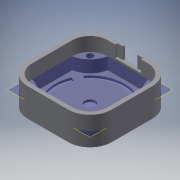
# Autodesk Inventor part: Oberbau
Saved by Autodesk Inventor 2018 (Build 220112000, 112)
## iProperties
Created: 2021-11-17
Part Number: Oberbau
Material: Generisch
Document SubType Name: Modeling
Designer: Markus
Density: 1 g/cm^3
Appearance: Vorgabe
Mass: 18.0219 g
Surface Area: 146.807 cm^2
Volume: 18.0219 cm^3
Author: Markus
Autodesk Inventor part; units mm, degrees
ref_plane "YZ Plane" through (0, 0, 0) normal (1, 0, 0) x (0, 1, 0)
ref_plane "XZ Plane" through (0, 0, 0) normal (0, 1, 0) x (-1, 0, 0)
ref_plane "XY Plane" through (0, 0, 0) normal (0, 0, 1) x (1, 0, 0)
sketch "Skizze1" plane through (0, 0, 0) normal (0, 0, 1) x (1, 0, 0)
  line L0 (-26, -14) -> (-26, 14)
  arc A0 (-14, 26) -> (-26, 14) centre (-14, 14) ccw
  line L1 (-14, 26) -> (14, 26)
  arc A1 (26, 14) -> (14, 26) centre (14, 14) ccw
  line L2 (26, 14) -> (26, -14)
  arc A2 (14, -26) -> (26, -14) centre (14, -14) ccw
  line L3 (14, -26) -> (-14, -26)
  arc A3 (-26, -14) -> (-14, -26) centre (-14, -14) ccw
  circle A4 centre (-7.42, 8.73) radius 0.55
  circle A5 centre (-7.42, 11.27) radius 0.55
  circle A6 centre (-3, 10.4) radius 0.4
  circle A7 centre (7.82, 11.27) radius 0.55
  circle A8 centre (7.82, 8.73) radius 0.55
  circle A9 centre (-2.5, 7) radius 0.5
  circle A10 centre (-7.42, 6.19) radius 0.55
  circle A11 centre (7.82, 6.19) radius 0.55
  circle A12 centre (2.5, 7) radius 0.5
  circle A13 centre (-7.42, 3.65) radius 0.55
  circle A14 centre (7.82, 3.65) radius 0.55
  circle A15 centre (0, -7.5) radius 0.5
  circle A16 centre (-2.5, -7.5) radius 0.5
  circle A17 centre (-7.42, -3.97) radius 0.55
  circle A18 centre (2.5, -7.5) radius 0.5
  circle A19 centre (-7.42, 1.11) radius 0.55
  circle A20 centre (-7.42, -1.43) radius 0.55
  circle A21 centre (7.82, -1.43) radius 0.55
  circle A22 centre (7.82, -3.97) radius 0.55
  circle A23 centre (7.82, 1.11) radius 0.55
  circle A24 centre (7.82, 23.97) radius 0.55
  circle A25 centre (7.82, 21.43) radius 0.55
  circle A26 centre (-7.42, 21.43) radius 0.55
  circle A27 centre (-3, 20.56) radius 0.4
  circle A28 centre (-7.42, 23.97) radius 0.55
  circle A29 centre (-7.42, 16.35) radius 0.55
  circle A30 centre (-7.42, 18.89) radius 0.55
  circle A31 centre (7.82, 18.89) radius 0.55
  circle A32 centre (7.82, 16.35) radius 0.55
  circle A33 centre (7.82, 13.81) radius 0.55
  circle A34 centre (-7.42, 13.81) radius 0.55
  circle A35 centre (20.37, 20.4) radius 1.6
  circle A36 centre (20.37, -20.34) radius 1.6
  circle A37 centre (-20.35, -20.31) radius 1.6
  circle A38 centre (-20.35, 20.4) radius 1.6
  line L4 (14, 29.080663) -> (-14, 29.080663)
  arc A39 (-14, 29.080663) -> (-29.080663, 14) centre (-14, 14) ccw
  line L5 (-29.080663, 14) -> (-29.080663, -14)
  arc A40 (-29.080663, -14) -> (-14, -29.080663) centre (-14, -14) ccw
  line L6 (-14, -29.080663) -> (14, -29.080663)
  arc A41 (14, -29.080663) -> (29.080663, -14) centre (14, -14) ccw
  line L7 (29.080663, -14) -> (29.080663, 14)
  arc A42 (29.080663, 14) -> (14, 29.080663) centre (14, 14) ccw
  line L8 (-14, -26.281068) -> (14, -26.281068)
  arc A43 (14, -26.281068) -> (26.281068, -14) centre (14, -14) ccw
  line L9 (26.281068, -14) -> (26.281068, 14)
  arc A44 (26.281068, 14) -> (14, 26.281068) centre (14, 14) ccw
  line L10 (14, 26.281068) -> (-14, 26.281068)
  arc A45 (-14, 26.281068) -> (-26.281068, 14) centre (-14, 14) ccw
  line L11 (-26.281068, 14) -> (-26.281068, -14)
  arc A46 (-26.281068, -14) -> (-14, -26.281068) centre (-14, -14) ccw
  point P0 (0, 0)
  constraints: 16 end point, 16 point on circle, 8 centre point, 14 other
extrude "Extrusion1" add sketch "Skizze1" against normal blind 10 contours A42 L7 A41 L6 A40 L5 A39 L4
ref_plane "Arbeitsebene1" through (0, 0, -1.6) normal (0, 0, -1) x (-1, 0, 0)
sketch "Skizze3 outline for Extrusion2" plane through (0, 0, -1.6) normal (0, 0, -1) x (-1, 0, 0)
  arc A0 (26.281068, -14) -> (14, -26.281068) centre (29.125158, -29.125158) ccw
  arc A1 (14, -26.281068) -> (26.281068, -14) centre (14, -14) ccw
  circle A2 centre (20.35, -20.31) radius 2.25
  arc A3 (-26.281068, -14) -> (-14, -26.281068) centre (-14, -14) ccw
  arc A4 (-14, -26.281068) -> (-26.281068, -14) centre (-29.125083, -29.125083) ccw
  circle A5 centre (-20.37, -20.34) radius 2.25
  arc A6 (-26.281068, 14) -> (-14, 26.281068) centre (-29.124991, 29.124991) ccw
  arc A7 (-14, 26.281068) -> (-26.281068, 14) centre (-14, 14) ccw
  circle A8 centre (-20.37, 20.4) radius 2.25
  arc A9 (14, 26.281068) -> (26.281068, 14) centre (29.114115, 29.114115) ccw
  arc A10 (26.281068, 14) -> (14, 26.281068) centre (14, 14) ccw
  circle A11 centre (20.35, 20.4) radius 2.25
extrude "Extrusion2" add sketch "Skizze3 outline for Extrusion2" along normal up to surface (8.4 mm away)
sketch "Skizze2" plane through (0, 0, -10) normal (0, 0, -1) x (-1, 0, 0)
  line L0 (14, 29.080663) -> (-14, 29.080663)
  arc A0 (-14, 29.080663) -> (-29.080663, 14) centre (-14, 14) ccw
  line L1 (-29.080663, 14) -> (-29.080663, -14)
  arc A1 (-29.080663, -14) -> (-14, -29.080663) centre (-14, -14) ccw
  line L2 (-14, -29.080663) -> (14, -29.080663)
  arc A2 (14, -29.080663) -> (29.080663, -14) centre (14, -14) ccw
  line L3 (29.080663, -14) -> (29.080663, 14)
  arc A3 (29.080663, 14) -> (14, 29.080663) centre (14, 14) ccw
  circle A4 centre (0, 0) radius 3.5
  circle A5 centre (0, 0) radius 3.5
  circle A6 centre (0, 0) radius 3.65
  point P0 (0, 0)
  dimension "d12" = 0.15
  constraints: 1 centre point
  measures "d12" radial gap between concentric circles of A4 A6
extrude "Extrusion3" add sketch "Skizze2" along normal blind 1.5 contours A3 L3 A2 L2 A1 L1 A0 L0
sketch "Skizze4" plane through (0, 0, 0) normal (0, 0, 1) x (1, 0, 0)
  line L0 (14, 29.080663) -> (-14, 29.080663)
  arc A0 (-14, 29.080663) -> (-29.080663, 14) centre (-14, 14) ccw
  line L1 (-29.080663, 14) -> (-29.080663, -14)
  arc A1 (-29.080663, -14) -> (-14, -29.080663) centre (-14, -14) ccw
  line L2 (-14, -29.080663) -> (14, -29.080663)
  arc A2 (14, -29.080663) -> (29.080663, -14) centre (14, -14) ccw
  line L3 (29.080663, -14) -> (29.080663, 14)
  arc A3 (29.080663, 14) -> (14, 29.080663) centre (14, 14) ccw
  arc A4 (14, -26.281068) -> (26.281068, -14) centre (14, -14) ccw
  line L4 (14, -26.281068) -> (-14, -26.281068)
  arc A5 (-26.281068, -14) -> (-14, -26.281068) centre (-14, -14) ccw
  line L5 (-26.281068, -14) -> (-26.281068, 14)
  arc A6 (-14, 26.281068) -> (-26.281068, 14) centre (-14, 14) ccw
  line L6 (-14, 26.281068) -> (14, 26.281068)
  arc A7 (26.281068, 14) -> (14, 26.281068) centre (14, 14) ccw
  line L7 (26.281068, 14) -> (26.281068, -14)
  line L8 (14, 29.080663) -> (-14, 29.080663)
  arc A8 (-14, 29.080663) -> (-29.080663, 14) centre (-14, 14) ccw
  line L9 (-29.080663, 14) -> (-29.080663, -14)
  arc A9 (-29.080663, -14) -> (-14, -29.080663) centre (-14, -14) ccw
  line L10 (-14, -29.080663) -> (14, -29.080663)
  arc A10 (14, -29.080663) -> (29.080663, -14) centre (14, -14) ccw
  line L11 (29.080663, -14) -> (29.080663, 14)
  arc A11 (29.080663, 14) -> (14, 29.080663) centre (14, 14) ccw
  point P0 (0, 0)
extrude "Extrusion4" add sketch "Skizze4" along normal blind 1.5
sketch "Skizze5" plane through (0, 0, 1.5) normal (0, 0, 1) x (1, 0, 0)
  line L0 (-3.62, 24.2) -> (-3.62, 28.75)
  line L1 (3.78, 24.2) -> (3.78, 28.75)
  line L2 (-3.62, 28.75) -> (-3.62, 29.080663)
  line L3 (14, 29.080663) -> (-14, 29.080663)
  line L4 (3.78, 28.75) -> (3.78, 29.080663)
  line L5 (3.78, 29.080663) -> (-3.62, 29.080663)
  line L6 (-14, 26) -> (14, 26)
  line L7 (-3.62, 26) -> (3.78, 26)
  line L8 (14, 29.080663) -> (-14, 29.080663)
  arc A0 (-14, 29.080663) -> (-29.080663, 14) centre (-14, 14) ccw
  line L9 (-29.080663, 14) -> (-29.080663, -14)
  arc A1 (-29.080663, -14) -> (-14, -29.080663) centre (-14, -14) ccw
  line L10 (-14, -29.080663) -> (14, -29.080663)
  arc A2 (14, -29.080663) -> (29.080663, -14) centre (14, -14) ccw
  line L11 (29.080663, -14) -> (29.080663, 14)
  arc A3 (29.080663, 14) -> (14, 29.080663) centre (14, 14) ccw
  line L12 (-4.92, 29.080663) -> (5.08, 29.080663)
  line L13 (5.08, 29.080663) -> (5.08, 26)
  line L14 (5.08, 26) -> (-4.92, 26)
  line L15 (-4.92, 26) -> (-4.92, 29.080663)
  line L16 (14, -26.281068) -> (-14, -26.281068)
  arc A4 (-26.281068, -14) -> (-14, -26.281068) centre (-14, -14) ccw
  line L17 (-26.281068, -14) -> (-26.281068, 14)
  arc A5 (-14, 26.281068) -> (-26.281068, 14) centre (-14, 14) ccw
  line L18 (-14, 26.281068) -> (14, 26.281068)
  arc A6 (26.281068, 14) -> (14, 26.281068) centre (14, 14) ccw
  line L19 (26.281068, 14) -> (26.281068, -14)
  arc A7 (14, -26.281068) -> (26.281068, -14) centre (14, -14) ccw
  line L20 (14, 29.080663) -> (-14, 29.080663)
  arc A8 (-14, 29.080663) -> (-29.080663, 14) centre (-14, 14) ccw
  line L21 (-29.080663, 14) -> (-29.080663, -14)
  arc A9 (-29.080663, -14) -> (-14, -29.080663) centre (-14, -14) ccw
  line L22 (-14, -29.080663) -> (14, -29.080663)
  arc A10 (14, -29.080663) -> (29.080663, -14) centre (14, -14) ccw
  line L23 (29.080663, -14) -> (29.080663, 14)
  arc A11 (29.080663, 14) -> (14, 29.080663) centre (14, 14) ccw
  point P0 (0, 0)
  point P1 (-4.12, 26)
  point P2 (-4.12, 29.080663)
  point P3 (4.28, 26)
  point P4 (4.28, 29.080663)
  dimension "d36" = 10
  constraints: 16 end point, 9 point on line, 3 parallel, 2 perpendicular, 1 horizontal, 1 vertical
  measures "d36" distance between parallel lines of L15 L13
extrude "Extrusion5" add sketch "Skizze5" along normal blind 8 contours L18 A5 L17 A4 L16 A7 L19 A6 L13 L3 A3 L11 A2 L10 A1 L9 A0 L15
sketch "Skizze6" plane through (0, 0, 9.5) normal (0, 0, 1) x (1, 0, 0)
  line L0 (8.97, 27.81) -> (8.97, -5.21)
  line L1 (-8.81, 27.81) -> (8.97, 27.81)
  line L2 (-8.81, -5.21) -> (-8.81, 27.81)
  line L3 (8.97, -5.21) -> (-8.81, -5.21)
  circle A0 centre (-7.55, -3.94) radius 0.530308
  circle A1 centre (-7.55, -1.4) radius 0.530308
  circle A2 centre (-7.55, 1.14) radius 0.530308
  circle A3 centre (-7.55, 3.68) radius 0.530308
  circle A4 centre (-7.55, 6.22) radius 0.530308
  circle A5 centre (-7.55, 8.76) radius 0.530308
  circle A6 centre (-7.55, 11.3) radius 0.530308
  circle A7 centre (-7.55, 13.84) radius 0.530308
  circle A8 centre (-7.55, 16.38) radius 0.530308
  circle A9 centre (-7.55, 18.92) radius 0.530308
  circle A10 centre (-7.55, 21.46) radius 0.530308
  circle A11 centre (-7.55, 24) radius 0.530308
  circle A12 centre (7.7, -3.94) radius 0.530308
  circle A13 centre (7.7, -1.4) radius 0.530308
  circle A14 centre (7.7, 1.14) radius 0.530308
  circle A15 centre (7.7, 3.68) radius 0.530308
  circle A16 centre (7.7, 6.22) radius 0.530308
  circle A17 centre (7.7, 8.76) radius 0.530308
  circle A18 centre (7.7, 11.3) radius 0.530308
  circle A19 centre (7.7, 13.84) radius 0.530308
  circle A20 centre (7.7, 16.38) radius 0.530308
  circle A21 centre (7.7, 18.92) radius 0.530308
  circle A22 centre (7.7, 21.46) radius 0.530308
  circle A23 centre (7.7, 24) radius 0.530308
  point P0 (0, 0)
extrude "Extrusion6" cut sketch "Skizze6" against normal up to surface (8 mm away)
sketch "Skizze7" plane through (0, 0, -11.5) normal (0, 0, -1) x (-1, 0, 0)
  circle A0 centre (0, 0) radius 22.5
  circle A1 centre (0, 0) radius 24
  circle A2 centre (0, 0) radius 21
  dimension "d23" = 45
  dimension "d24" = 1.5
  dimension "d25" = 1.5
  constraints: 3 centre point, 1 coincident
  measures "d23" diameter of A0
  measures "d24" radial gap between concentric circles of A0 A1
  measures "d25" radial gap between concentric circles of A0 A2
extrude "Extrusion7" cut sketch "Skizze7" against normal blind 5.75 contours A0 | A1
sketch "Skizze8" plane through (0, 0, -11.5) normal (0, 0, -1) x (-1, 0, 0)
  circle A0 centre (8, -21) radius 1.666667
  circle A1 centre (-8, -21) radius 1.666667
  circle A2 centre (-20, -10.4) radius 1.666667
  circle A3 centre (-21.8, 5.5) radius 1.666667
  circle A4 centre (19.9, -10.4) radius 1.666667
  circle A5 centre (21.8, 5.5) radius 1.666667
  circle A6 centre (12.7, 18.6) radius 1.666667
  circle A7 centre (-12.7, 18.6) radius 1.666667
  line L0 (14, 29.080663) -> (-14, 29.080663)
  arc A8 (-14, 29.080663) -> (-29.080663, 14) centre (-14, 14) ccw
  line L1 (-29.080663, 14) -> (-29.080663, -14)
  arc A9 (-29.080663, -14) -> (-14, -29.080663) centre (-14, -14) ccw
  line L2 (-14, -29.080663) -> (14, -29.080663)
  arc A10 (14, -29.080663) -> (29.080663, -14) centre (14, -14) ccw
  line L3 (29.080663, -14) -> (29.080663, 14)
  arc A11 (29.080663, 14) -> (14, 29.080663) centre (14, 14) ccw
  circle A12 centre (0, 0) radius 24
  circle A13 centre (0, 0) radius 21
  line L4 (3, -23.811762) -> (2.625, -20.835292)
  circle A14 centre (0, 0) radius 21
  line L5 (0, -24) -> (0, -21)
  line L6 (-2.625, -20.835292) -> (-3, -23.811762)
  circle A15 centre (0, 0) radius 24
  dimension "d29" = 3
  dimension "d30" = 3
  constraints: 6 end point, 6 point on circle, 3 line through centre, 1 vertical
  measures "d29" distance from line of L5 L6.end
  measures "d30" distance from line of L5 L4.start
extrude "Extrusion8" add sketch "Skizze8" against normal up to surface (1.5 mm away) contours L4 A12 L5 A13 | L5 A12 L6 A13
pattern_circular "Runde Anordnung1" count 3 over 360 about axis through (0, 0, -11.5) along (0, 0, 1) of "Extrusion8"
sketch "Skizze9" plane through (0, 0, 1.5) normal (0, 0, 1) x (1, 0, 0)
  line L0 (5.08, 27.81) -> (5.08, 29.080663)
  line L1 (5.08, 29.080663) -> (-4.92, 29.080663)
  line L2 (-4.92, 29.080663) -> (-4.92, 27.81)
  line L3 (-8.81, 27.81) -> (-4.92, 27.81)
  line L4 (-8.81, 26.281068) -> (-8.81, 27.81)
  line L5 (-8.81, 26.281068) -> (8.97, 26.281068)
  line L6 (8.97, 27.81) -> (8.97, 26.281068)
  line L7 (5.08, 27.81) -> (8.97, 27.81)
  point P0 (0, 0)
extrude "Extrusion9" cut sketch "Skizze9" against normal blind 1.7
sketch "Skizze10" plane through (0, 0, 9.5) normal (0, 0, 1) x (1, 0, 0)
  line L0 (8.97, 27.81) -> (8.97, 26.281068)
  line L1 (8.97, 26.281068) -> (14, 26.281068)
  arc A0 (26.281068, 14) -> (14, 26.281068) centre (14, 14) ccw
  line L2 (26.281068, 14) -> (26.281068, -14)
  arc A1 (14, -26.281068) -> (26.281068, -14) centre (14, -14) ccw
  line L3 (14, -26.281068) -> (-14, -26.281068)
  arc A2 (-26.281068, -14) -> (-14, -26.281068) centre (-14, -14) ccw
  line L4 (-26.281068, -14) -> (-26.281068, 14)
  arc A3 (-14, 26.281068) -> (-26.281068, 14) centre (-14, 14) ccw
  line L5 (-14, 26.281068) -> (-8.81, 26.281068)
  line L6 (-8.81, 26.281068) -> (-8.81, 27.81)
  line L7 (-8.81, 27.81) -> (-4.92, 27.81)
  line L8 (-4.92, 27.81) -> (-4.92, 29.080663)
  line L9 (-4.92, 29.080663) -> (-14, 29.080663)
  arc A4 (-14, 29.080663) -> (-29.080663, 14) centre (-14, 14) ccw
  line L10 (-29.080663, 14) -> (-29.080663, -14)
  arc A5 (-29.080663, -14) -> (-14, -29.080663) centre (-14, -14) ccw
  line L11 (-14, -29.080663) -> (14, -29.080663)
  arc A6 (14, -29.080663) -> (29.080663, -14) centre (14, -14) ccw
  line L12 (29.080663, -14) -> (29.080663, 14)
  arc A7 (29.080663, 14) -> (14, 29.080663) centre (14, 14) ccw
  line L13 (14, 29.080663) -> (5.08, 29.080663)
  line L14 (5.08, 29.080663) -> (5.08, 27.81)
  line L15 (5.08, 27.81) -> (8.97, 27.81)
  point P0 (0, 0)
extrude "Extrusion10" cut sketch "Skizze10" against normal blind 1.5
